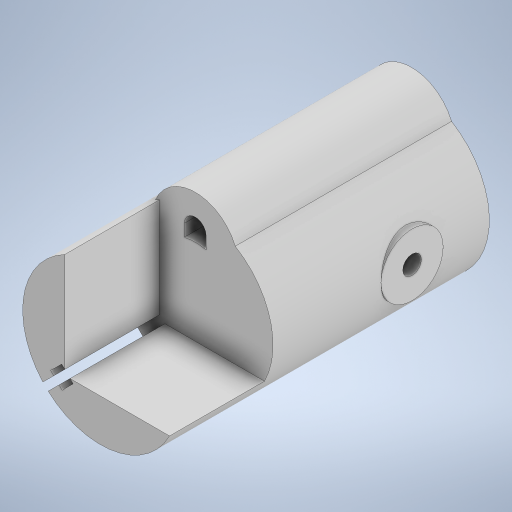
# Autodesk Inventor part: LandingFoot2
Saved by Autodesk Inventor 2023 (Build 270158000, 158)
## iProperties
Created: 2023-01-25
Part Number: LandingFoot2
Material: Generic
Document SubType Name: Modeling
Designer: chase
Density: 1 g/cm^3
Appearance: Default
Author: chase
Autodesk Inventor part; units mm, degrees
ref_plane "YZ Plane" through (0, 0, 0) normal (1, 0, 0) x (0, 1, 0)
sketch "Sketch1" plane through (0, 0, 0) normal (0, 0, 1) x (1, 0, 0)
  circle A0 centre (0, 0) radius 12.5
  dimension "d0" = 25
  constraints: 1 centre point, 1 coincident
  measures "d0" diameter of A0
extrude "Extrusion1" add sketch "Sketch1" against normal blind 50
sketch "Sketch2" plane through (0, 0, -50) normal (0, 0, -1) x (-1, 0, 0)
  circle A0 centre (0, 0) radius 8.075
  dimension "d3" = 16.15
  constraints: 1 centre point, 1 coincident
  measures "d3" diameter of A0
extrude "Extrusion2" cut sketch "Sketch2" against normal blind 25.4
sketch "Sketch3" plane through (0, 0, 0) normal (0, 0, 1) x (1, 0, 0)
  circle A0 centre (0, 0) radius 12.5
  line L0 (0, 12.5) -> (0, 0) construction
  line L1 (-4.4548, -2.6163) -> (-9.7581, -7.9196)
  line L2 (-9.7581, -7.9196) -> (-7.955, -9.7227)
  line L3 (-7.9196, -9.7581) -> (-2.6163, -4.4548)
  line L4 (-9.7227, -7.955) -> (-7.9196, -9.7581)
  line L5 (-6.2225, -4.3841) -> (-4.3841, -6.2225)
  line L6 (-7.9903, -6.1518) -> (-6.1518, -7.9903)
  line L7 (-8.4146, -9.2631) -> (-6.6468, -7.4953)
  line L8 (-9.2631, -8.4146) -> (-7.4953, -6.6468)
  line L9 (-4.4548, -2.6163) -> (-2.6517, -4.4194)
  line L10 (-4.879, -5.7276) -> (-4.5255, -5.374)
  line L11 (-5.7276, -4.879) -> (-5.374, -4.5255)
  line L12 (-5.374, -4.5255) -> (-4.5255, -5.374)
  line L13 (-4.9497, -4.9497) -> (-3.5355, -3.5355)
  line L14 (-5.2679, -4.6315) -> (-3.8537, -3.2173)
  line L15 (-4.6315, -5.2679) -> (-3.2173, -3.8537)
  line L16 (-4.4194, -2.6517) -> (-2.6163, -4.4548)
  line L17 (-4.879, -5.7276) -> (11.1106, -5.7276)
  line L18 (-5.7276, -4.879) -> (-5.7276, 11.1106)
  line L19 (0, 0) -> (-3.5355, -3.5355) construction
  line L20 (-4.9497, -4.9497) -> (-8.8388, -8.8388) construction
  point P0 (-6.1872, -4.4194)
  point P1 (-7.955, -6.1872)
  point P2 (-6.1872, -7.955)
  point P3 (-4.4194, -6.1872)
  point P4 (-5.7276, -3.8891)
  point P5 (-3.8891, -5.7276)
  point P6 (-9.7101, -7.8717)
  point P7 (-9.2529, -8.4044)
  point P8 (-8.4044, -9.2529)
  point P9 (-8.8388, -8.8388)
  point P10 (-7.8717, -9.7101)
  dimension "d44" = 0.9
  dimension "d45" = 0.45
  dimension "d47" = 1.2
  dimension "d48" = 0.6
  dimension "d49" = 2.5
  dimension "d50" = 2.5
  dimension "d51" = 2.5
  dimension "d52" = 0.5
  dimension "d53" = 2.6
  dimension "d54" = 1.3
  constraints: 42 end point, 4 point on line, 1 collinear, 1 vertical, 3 other
  measures "d44" distance between parallel lines of L15 L14
  measures "d45" distance between parallel lines of L13 L14
  measures "d47" distance between parallel lines of L7 L8
  measures "d48" distance between parallel lines of L7 L20
  measures "d49" distance between parallel lines of L6 L5
  measures "d50" distance between parallel lines of L2 L6
  measures "d51" distance between parallel lines of L5 L9
  measures "d52" distance between parallel lines of L5 L12
  measures "d53" distance between parallel lines of L3 L1
  measures "d54" distance between parallel lines of L3 L13
sketch "Sketch4" plane through (0, 0, -50) normal (0, 0, -1) x (-1, 0, 0)
  arc A0 (6.4283, 10.7204) -> (-6.4283, 10.7204) centre (0, 8.075) ccw
  arc A1 (1.5, 7.9345) -> (-1.5, 7.9345) centre (0, 0) ccw
  circle A2 centre (0, 0) radius 12.5
  point P0 (0, 8.075)
  dimension "d17" = 12.8567
  dimension "d18" = 6.4283
  constraints: 8 point on circle, 3 centre point
  measures "d17" distance of A0.start A0.end
  measures "d18" horizontal distance of A0.start point (0, 8.075)
sketch "Sketch5" plane through (0, 0, -50) normal (0, 0, -1) x (-1, 0, 0)
  circle A0 centre (0, 9.825) radius 1.75
  line L0 (-1.75, 9.825) -> (-1.75, 7.8831)
  line L1 (1.75, 9.825) -> (1.75, 7.8831)
  circle A1 centre (0, 0) radius 8.075
  circle A2 centre (0, 0) radius 8.075 projected
  point P0 (-1.75, 7.8831)
  point P1 (1.75, 7.8831)
  dimension "d21" = 3.5
  dimension "d22" = 16.15
  dimension "d63" = 0
  constraints: 4 end point, 4 point on circle, 2 centre point, 1 coincident, 1 parallel, 1 tangent, 1 vertical
  measures "d21" diameter of A0
  measures "d22" diameter of A1
  measures "d63" horizontal distance of point (0, 0) A0.centre
ref_plane "Work Plane1" through (12.5, 0, 0) normal (1, 0, 0) x (0, 0, -1)
ref_plane "Work Plane2" through (-12.5, 0, 0) normal (1, 0, 0) x (0, 0, -1)
sketch "Sketch6" plane through (12.5, 0, 0) normal (1, 0, 0) x (0, 0, -1)
  circle A0 centre (37.5833, 0) radius 5
  point P0 (0, 0)
  constraints: 1 centre point
extrude "Extrusion6" add sketch "Sketch6" against normal up to surface (25 mm away)
sketch "Sketch7" plane through (12.5, 0, 0) normal (1, 0, 0) x (0, 0, -1)
  arc A0 (42.5833, 0) -> (32.5833, 0) centre (37.5833, 0) ccw projected
  circle A1 centre (37.5833, 0) radius 1.5
  point P0 (0, 0)
  dimension "d29" = 3
  constraints: 1 centre point, 1 coincident
  measures "d29" diameter of A1
extrude "Extrusion7" cut sketch "Sketch7" against normal up to surface (25 mm away)
sketch "Sketch8" plane through (0, 0, -50) normal (0, 0, -1) x (-1, 0, 0)
  arc A0 (8.075, 0) -> (8.075, 0) centre (0, 0) ccw projected
  circle A1 centre (0, 0) radius 8.075
  point P0 (1.5, 7.9345)
  point P1 (-1.5, 7.9345)
  constraints: 1 centre point, 1 coincident
extrude "Extrusion9" cut sketch "Sketch3" against normal blind 15.24 contours A0 L17 L3 L16 L9 L1 L18 | L1 L9 L14 L12 L11 L18 | L17 L10 L12 L15 L9 L16 L3 | L8 L6 L7 A0 | A0 L2 L8 | L1 L5 L3 L6 | L11 L12 L10 L5 | L7 L2 A0 | L9 L13 L12 L14 | L15 L12 L13 L9
extrude "Extrusion10" add sketch "Sketch4" against normal up to surface (34.76 mm away) contours A2 A0
extrude "Extrusion11" cut sketch "Sketch5" against normal through all contours A0 | L1 A1 A0 | A0 A1 L0
extrude "Extrusion12" cut sketch "Sketch8" against normal up to surface (25.4 mm away)
equation "\"d45\" = 0.5 * d44"
equation "\"d48\" = 0.5 * d47"
equation "\"d54\" = 0.5 * d53"
equation "\"d18\" = 0.5 * d17"
body "Solid1"
